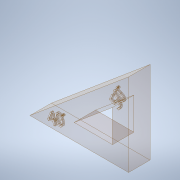
# Autodesk Inventor part: 40-50-6in-Template
Saved by Autodesk Inventor 2020.2 (Build 242310000, 310)
## iProperties
Created: 2020-01-27
Part Number: 40-50-6in-Template
Material: PET Plastic
Document SubType Name: Modeling
Designer: robst
Density: 1.541 g/cm^3
Appearance: Polycarbonate - Smoked
Author: robst
Autodesk Inventor part; units mm, degrees
ref_plane "YZ Plane" through (0, 0, 0) normal (1, 0, 0) x (0, 1, 0)
ref_plane "XZ Plane" through (0, 0, 0) normal (0, 1, 0) x (-1, 0, 0)
ref_plane "XY Plane" through (0, 0, 0) normal (0, 0, 1) x (1, 0, 0)
sketch "Sketch1" plane through (0, 0, 0) normal (0, 0, 1) x (1, 0, 0)
  line L0 (0, 0) -> (116.7452, 97.9608)
  line L1 (0, 0) -> (152.4, 0) construction
  line L2 (116.7452, 97.9608) -> (116.7452, 0)
  line L3 (116.7452, 0) -> (0, 0)
  dimension "d0" = 152.4
  dimension "d1" = 40
  constraints: 8 end point, 1 equal length, 1 horizontal, 1 perpendicular, 1 vertical
  measures "d0" distance of L0.start L0.end
  measures "d1" angle of L1 L0
extrude "Extrusion1" add sketch "Sketch1" along normal mid plane 25.4
sketch "Sketch2" plane through (0, 0, 12.7) normal (0, 0, 1) x (1, 0, 0)
  line L0 (0, 0) -> (116.7452, 0) construction
  line L1 (0, 0) -> (116.7452, 42.4918) construction
  line L2 (116.7452, 0) -> (116.7452, 97.9608) construction
  line L3 (29.7312, 8.7075) -> (28.3096, 8.1901)
  line L4 (28.3096, 8.1901) -> (29.8021, 4.0895)
  line L5 (29.8021, 4.0895) -> (28.2644, 3.5299)
  line L6 (28.2644, 3.5299) -> (26.7719, 7.6304)
  line L7 (26.7719, 7.6304) -> (21.5012, 5.712)
  line L8 (21.5012, 5.712) -> (20.8887, 7.3948)
  line L9 (20.8887, 7.3948) -> (23.9884, 15.4886)
  line L10 (23.9884, 15.4886) -> (25.4584, 16.0236)
  line L11 (25.4584, 16.0236) -> (27.8414, 9.4763)
  line L12 (27.8414, 9.4763) -> (29.2631, 9.9938)
  line L13 (29.2631, 9.9938) -> (29.7312, 8.7075)
  line L14 (26.3037, 8.9166) -> (24.6071, 13.5781)
  line L15 (24.6071, 13.5781) -> (22.2902, 7.4559)
  line L16 (22.2902, 7.4559) -> (26.3037, 8.9166)
  spline S0 degree 2 poles (37.7558, 13.742) (38.9245, 10.5312) (38.1527, 6.8442) (36.2088, 6.1366) knots 0 0 0 1 2 2 2
  spline S1 degree 2 poles (36.2088, 6.1366) (34.2359, 5.4186) (31.2729, 7.812) (30.1289, 10.9551) knots 0 0 0 1 2 2 2
  spline S2 degree 2 poles (30.1289, 10.9551) (28.9532, 14.1852) (29.7321, 17.8529) (31.6856, 18.564) knots 0 0 0 1 2 2 2
  spline S3 degree 2 poles (31.6856, 18.564) (33.6488, 19.2785) (36.6224, 16.8561) (37.7558, 13.742) knots 0 0 0 1 2 2 2
  spline S4 degree 2 poles (37.0291, 9.3594) (37.0465, 10.0339) (36.5781, 11.9224) (36.1311, 13.1506) knots 0 0 0 1 2 2 2
  spline S5 degree 2 poles (36.1311, 13.1506) (35.6841, 14.3789) (34.8324, 16.117) (34.3689, 16.6382) knots 0 0 0 1 2 2 2
  spline S6 degree 2 poles (34.3689, 16.6382) (33.9053, 17.1595) (32.8352, 17.4819) (32.1679, 17.239) knots 0 0 0 1 2 2 2
  spline S7 degree 2 poles (32.1679, 17.239) (31.5005, 16.9961) (30.8686, 16.0542) (30.846, 15.3341) knots 0 0 0 1 2 2 2
  spline S8 degree 2 poles (30.846, 15.3341) (30.826, 14.6368) (31.3277, 12.7166) (31.7536, 11.5464) knots 0 0 0 1 2 2 2
  spline S9 degree 2 poles (31.7536, 11.5464) (32.2112, 10.2892) (32.9784, 8.6627) (33.4692, 8.0966) knots 0 0 0 1 2 2 2
  spline S10 degree 2 poles (33.4692, 8.0966) (33.9266, 7.5622) (35.0302, 7.2081) (35.7266, 7.4616) knots 0 0 0 1 2 2 2
  spline S11 degree 2 poles (35.7266, 7.4616) (36.3842, 7.7009) (37.0161, 8.6428) (37.0291, 9.3594) knots 0 0 0 1 2 2 2
  spline S12 degree 2 poles (38.4763, 17.6439) (37.9694, 17.4594) (36.9953, 17.9137) (36.815, 18.409) knots 0 0 0 1 2 2 2
  spline S13 degree 2 poles (36.815, 18.409) (36.6305, 18.9159) (37.0848, 19.89) (37.5916, 20.0745) knots 0 0 0 1 2 2 2
  spline S14 degree 2 poles (37.5916, 20.0745) (38.087, 20.2548) (39.0611, 19.8005) (39.2456, 19.2937) knots 0 0 0 1 2 2 2
  spline S15 degree 2 poles (39.2456, 19.2937) (39.4259, 18.7983) (38.9716, 17.8242) (38.4763, 17.6439) knots 0 0 0 1 2 2 2
  spline S16 degree 2 poles (37.9564, 19.0723) (37.7375, 18.9926) (37.8172, 18.7738) knots 0 0 0 1 1 1
  spline S17 degree 2 poles (37.8172, 18.7738) (37.8926, 18.5664) (38.1115, 18.6461) knots 0 0 0 1 1 1
  spline S18 degree 2 poles (38.1115, 18.6461) (38.3189, 18.7216) (38.2434, 18.9289) knots 0 0 0 1 1 1
  spline S19 degree 2 poles (38.2434, 18.9289) (38.1637, 19.1478) (37.9564, 19.0723) knots 0 0 0 1 1 1
  dimension "d4" = 20
  constraints: 2 end point, 1 point on line, 1 other
  measures "d4" angle of L1 L0
sketch "Sketch3" plane through (0, 0, 12.7) normal (0, 0, 1) x (1, 0, 0)
  line L0 (116.7452, 97.9608) -> (0, 0) construction
  line L1 (116.7452, 97.9608) -> (71.0653, 0) construction
  line L2 (0, 0) -> (116.7452, 0) construction
  line L3 (116.7452, 0) -> (116.7452, 97.9608) construction
  spline S0 degree 2 poles (104.4715, 66.1606) (105.3016, 65.7735) (106.4715, 64.5807) (106.7677, 63.8521) knots 0 0 0 1 2 2 2
  spline S1 degree 2 poles (106.7677, 63.8521) (107.0638, 63.1235) (106.9959, 61.395) (106.5784, 60.4996) knots 0 0 0 1 2 2 2
  spline S2 degree 2 poles (106.5784, 60.4996) (106.1956, 59.6787) (105.0838, 58.244) (104.5206, 57.7912) knots 0 0 0 1 2 2 2
  line L4 (104.5206, 57.7912) -> (102.8883, 58.5524)
  line L5 (102.8883, 58.5524) -> (102.9405, 58.6643)
  spline S3 degree 2 poles (102.9405, 58.6643) (103.1537, 58.7807) (103.7983, 59.2863) (104.1346, 59.6178) knots 0 0 0 1 2 2 2
  spline S4 degree 2 poles (104.1346, 59.6178) (104.5063, 60.0009) (105.0358, 60.6738) (105.2576, 61.1495) knots 0 0 0 1 2 2 2
  spline S5 degree 2 poles (105.2576, 61.1495) (105.4751, 61.6159) (105.5481, 62.6493) (105.3323, 63.136) knots 0 0 0 1 2 2 2
  spline S6 degree 2 poles (105.3323, 63.136) (105.122, 63.5861) (104.3471, 64.3108) (103.7314, 64.5979) knots 0 0 0 1 2 2 2
  spline S7 degree 2 poles (103.7314, 64.5979) (103.1158, 64.885) (102.1757, 64.9145) (101.7667, 64.7192) knots 0 0 0 1 2 2 2
  spline S8 degree 2 poles (101.7667, 64.7192) (101.3253, 64.5275) (100.6305, 63.6706) (100.3564, 63.0829) knots 0 0 0 1 2 2 2
  spline S9 degree 2 poles (100.3564, 63.0829) (100.0607, 62.4487) (99.6694, 61.0981) (99.575, 60.6766) knots 0 0 0 1 2 2 2
  line L6 (99.575, 60.6766) -> (93.6427, 63.4428)
  line L7 (93.6427, 63.4428) -> (96.5873, 69.7575)
  line L8 (96.5873, 69.7575) -> (97.9398, 69.1269)
  line L9 (97.9398, 69.1269) -> (95.6868, 64.2952)
  line L10 (95.6868, 64.2952) -> (98.7555, 62.8642)
  spline S10 degree 2 poles (98.7555, 62.8642) (98.8487, 63.1615) (99.073, 63.7155) (99.1774, 63.9394) knots 0 0 0 1 2 2 2
  spline S11 degree 2 poles (99.1774, 63.9394) (99.5906, 64.8255) (100.4495, 65.9125) (101.1395, 66.2721) knots 0 0 0 1 2 2 2
  spline S12 degree 2 poles (101.1395, 66.2721) (101.8339, 66.641) (103.4268, 66.6477) (104.4715, 66.1606) knots 0 0 0 1 2 2 2
  spline S13 degree 2 poles (106.4874, 75.963) (109.5841, 74.519) (111.6455, 71.3661) (110.7713, 69.4912) knots 0 0 0 1 2 2 2
  spline S14 degree 2 poles (110.7713, 69.4912) (109.884, 67.5884) (106.0964, 67.1857) (103.065, 68.5993) knots 0 0 0 1 2 2 2
  spline S15 degree 2 poles (103.065, 68.5993) (99.9496, 70.052) (97.9069, 73.1962) (98.7855, 75.0803) knots 0 0 0 1 2 2 2
  spline S16 degree 2 poles (98.7855, 75.0803) (99.6684, 76.9738) (103.484, 77.3635) (106.4874, 75.963) knots 0 0 0 1 2 2 2
  spline S17 degree 2 poles (109.0725, 72.3502) (108.6079, 72.8393) (106.9413, 73.8436) (105.7567, 74.396) knots 0 0 0 1 2 2 2
  spline S18 degree 2 poles (105.7567, 74.396) (104.5721, 74.9484) (102.7409, 75.5752) (102.0445, 75.616) knots 0 0 0 1 2 2 2
  spline S19 degree 2 poles (102.0445, 75.616) (101.3481, 75.6568) (100.3635, 75.128) (100.0633, 74.4844) knots 0 0 0 1 2 2 2
  spline S20 degree 2 poles (100.0633, 74.4844) (99.7632, 73.8408) (99.9824, 72.728) (100.4756, 72.2028) knots 0 0 0 1 2 2 2
  spline S21 degree 2 poles (100.4756, 72.2028) (100.9545, 71.6956) (102.6671, 70.6926) (103.7957, 70.1663) knots 0 0 0 1 2 2 2
  spline S22 degree 2 poles (103.7957, 70.1663) (105.0083, 69.6008) (106.7009, 68.9933) (107.4482, 68.94) knots 0 0 0 1 2 2 2
  spline S23 degree 2 poles (107.4482, 68.94) (108.1496, 68.8855) (109.1803, 69.4155) (109.4934, 70.0871) knots 0 0 0 1 2 2 2
  spline S24 degree 2 poles (109.4934, 70.0871) (109.7892, 70.7214) (109.57, 71.8343) (109.0725, 72.3502) knots 0 0 0 1 2 2 2
  spline S25 degree 2 poles (104.2378, 79.2315) (104.0098, 78.7426) (102.9998, 78.375) (102.5221, 78.5978) knots 0 0 0 1 2 2 2
  spline S26 degree 2 poles (102.5221, 78.5978) (102.0332, 78.8257) (101.6656, 79.8358) (101.8935, 80.3246) knots 0 0 0 1 2 2 2
  spline S27 degree 2 poles (101.8935, 80.3246) (102.1163, 80.8023) (103.1263, 81.17) (103.6152, 80.942) knots 0 0 0 1 2 2 2
  spline S28 degree 2 poles (103.6152, 80.942) (104.0929, 80.7192) (104.4606, 79.7092) (104.2378, 79.2315) knots 0 0 0 1 2 2 2
  spline S29 degree 2 poles (102.8601, 79.8739) (102.7617, 79.6628) (102.9728, 79.5644) knots 0 0 0 1 1 1
  spline S30 degree 2 poles (102.9728, 79.5644) (103.1728, 79.4711) (103.2712, 79.6822) knots 0 0 0 1 1 1
  spline S31 degree 2 poles (103.2712, 79.6822) (103.3645, 79.8822) (103.1645, 79.9754) knots 0 0 0 1 1 1
  spline S32 degree 2 poles (103.1645, 79.9754) (102.9534, 80.0739) (102.8601, 79.8739) knots 0 0 0 1 1 1
  dimension "d5" = 25
  constraints: 2 end point, 1 point on line, 1 other
  measures "d5" angle of L1 L3
extrude "Extrusion2" cut sketch "Sketch2" against normal blind 2.54
extrude "Extrusion3" cut sketch "Sketch3" against normal blind 2.54
sketch "Sketch4" plane through (0, 0, 12.7) normal (0, 0, 1) x (1, 0, 0)
  line L0 (52.3394, 19.05) -> (97.6952, 19.05)
  line L1 (97.6952, 19.05) -> (97.6952, 57.108)
  line L2 (97.6952, 57.108) -> (52.3394, 19.05)
  line L3 (0, 0) -> (116.7452, 0) projected
  line L4 (116.7452, 0) -> (116.7452, 97.9608) projected
  line L5 (116.7452, 97.9608) -> (0, 0) projected
  dimension "d10" = 19.05
  dimension "d11" = 19.05
  dimension "d12" = 19.05
  constraints: 6 end point, 3 parallel, 1 horizontal, 1 perpendicular
  measures "d10" distance between parallel lines of L0 L3
  measures "d11" distance between parallel lines of L1 L4
  measures "d12" distance between parallel lines of L2 L5
extrude "Extrusion4" cut sketch "Sketch4" against normal through all contours L2 L1 L0
body "Solid1"
